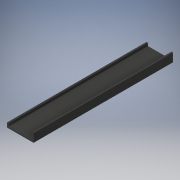
# Autodesk Inventor part: trocador1
Saved by Autodesk Inventor 2019.4 (Build 234330000, 330)
## iProperties
Created: 2020-04-10
Part Number: trocador1
Material: Ouro
Document SubType Name: Modeling
Designer: lucas
Density: 19.3 g/cm^3
Appearance: Liso - Preto
Author: lucas
Autodesk Inventor part; units mm, degrees
ref_plane "YZ Plane" through (0, 0, 0) normal (1, 0, 0) x (0, 1, 0)
ref_plane "XZ Plane" through (0, 0, 0) normal (0, 1, 0) x (-1, 0, 0)
ref_plane "XY Plane" through (0, 0, 0) normal (0, 0, 1) x (1, 0, 0)
sketch "Esboço1" plane through (0, 0, 0) normal (0, 0, 1) x (1, 0, 0)
  line L0 (0, 0) -> (190, 0)
  line L1 (190, 0) -> (190, 60)
  line L2 (190, 60) -> (180, 60)
  line L3 (180, 60) -> (180, 10)
  line L4 (180, 10) -> (10, 10)
  line L5 (10, 10) -> (10, 30)
  line L6 (10, 30) -> (0, 30)
  line L7 (0, 30) -> (0, 0)
  dimension "d0" = 190
  dimension "d1" = 10
  dimension "d2" = 60
  dimension "d3" = 10
  dimension "d4" = 10
  dimension "d5" = 30
  constraints: 16 end point, 7 perpendicular, 1 horizontal
  measures "d0" distance of L0.start L0.end
  measures "d1" distance between parallel lines of L5 L7
  measures "d2" distance of L0.end L1.end
  measures "d3" distance between parallel lines of L1 L3
  measures "d4" distance between parallel lines of L0 L4
  measures "d5" distance between parallel lines of L0 L6
extrude "Extrusão1" add sketch "Esboço1" along normal blind 1000
